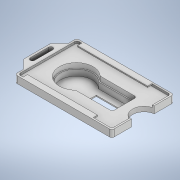
# Autodesk Inventor part: Badge
Saved by Autodesk Inventor 2020 (Build 240168000, 168)
## iProperties
Created: 2019-12-22
Part Number: Badge
Material: Generic
Document SubType Name: Modeling
Designer: user
Density: 1 g/cm^3
Appearance: Default
Author: user
## iProperties of the stored document _3DPrint.ipt
Created: 2019-12-23
Part Number: _3DPrint
Material: Generic
Document SubType Name: Modeling
Designer: user
Density: 1 g/cm^3
Appearance: Default
Author: user
Autodesk Inventor part; units mm, degrees
ref_plane "YZ Plane" through (0, 0, 0) normal (1, 0, 0) x (0, 1, 0)
ref_plane "XZ Plane" through (0, 0, 0) normal (0, 1, 0) x (-1, 0, 0)
ref_plane "XY Plane" through (0, 0, 0) normal (0, 0, 1) x (1, 0, 0)
sketch "Sketch1" plane through (0, 0, 0) normal (0, 1, 0) x (-1, 0, 0)
  line L0 (8.4719, 24.6226) -> (-76.3226, 24.6226)
  line L1 (-76.3281, -32.1774) -> (8.4719, -32.1774)
  line L2 (10.4719, 16.6226) -> (17.8861, 9.2084)
  line L3 (18.4719, 7.7942) -> (18.4719, -15.3489)
  line L4 (17.8861, -16.7632) -> (10.4719, -24.1774)
  line L5 (12.4719, 4.6226) -> (12.4719, -12.1774)
  line L6 (16.4719, -12.1774) -> (16.4719, 4.6226)
  arc A0 (14.4719, -14.1774) -> (16.4719, -12.1774) centre (14.4719, -12.1774) ccw
  arc A1 (12.4719, -12.1774) -> (14.4719, -14.1774) centre (14.4719, -12.1774) ccw
  arc A2 (14.4719, 6.6226) -> (12.4719, 4.6226) centre (14.4719, 4.6226) ccw
  arc A3 (16.4719, 4.6226) -> (14.4719, 6.6226) centre (14.4719, 4.6226) ccw
  arc A4 (-78.3281, -14.1774) -> (-78.3226, 6.6226) centre (-79.4686, -3.7771) ccw
  circle A5 centre (-17.3753, -3.7774) radius 15.5
  line L7 (-61.5377, 5.4726) -> (-61.5377, -13.0274)
  line L8 (-59.5377, -15.0274) -> (-28.0377, -15.0274)
  line L9 (-28.0377, 7.4726) -> (-59.5377, 7.4726)
  arc A6 (-61.5377, -13.0274) -> (-59.5377, -15.0274) centre (-59.5377, -13.0274) ccw
  arc A7 (-59.5377, 7.4726) -> (-61.5377, 5.4726) centre (-59.5377, 5.4726) ccw
  line L10 (-31.4377, 0.4726) -> (-56.9377, 0.4726)
  line L11 (-56.9377, 0.4726) -> (-56.9377, -8.0274)
  line L12 (-56.9377, -8.0274) -> (-31.4377, -8.0274)
  line L13 (-31.4377, -8.0274) -> (-31.4377, 0.4726)
  line L14 (-78.3226, 6.6226) -> (-78.3226, 22.6226)
  line L15 (-78.3281, -14.1774) -> (-78.3281, -30.1774)
  line L16 (6.9737, 23.1226) -> (-74.8281, 23.1226)
  line L17 (-74.8281, -30.6774) -> (6.9737, -30.6774)
  line L18 (8.9737, -28.6774) -> (8.9737, 21.1226)
  line L19 (-76.8281, 21.1226) -> (-76.8281, 6.3469)
  line L20 (-76.8281, -28.6774) -> (-76.8281, -13.901)
  line L21 (10.4719, 22.6226) -> (10.4719, 16.6226)
  line L22 (10.4719, -24.1774) -> (10.4719, -30.1774)
  arc A8 (-78.3281, -30.1774) -> (-76.3281, -32.1774) centre (-76.3281, -30.1774) ccw
  arc A9 (-76.8281, -28.6774) -> (-74.8281, -30.6774) centre (-74.8281, -28.6774) ccw
  arc A10 (-74.8281, 23.1226) -> (-76.8281, 21.1226) centre (-74.8281, 21.1226) ccw
  arc A11 (-76.3226, 24.6226) -> (-78.3226, 22.6226) centre (-76.3226, 22.6226) ccw
  arc A12 (10.4719, 22.6226) -> (8.4719, 24.6226) centre (8.4719, 22.6226) ccw
  arc A13 (8.9737, 21.1226) -> (6.9737, 23.1226) centre (6.9737, 21.1226) ccw
  arc A14 (6.9737, -30.6774) -> (8.9737, -28.6774) centre (6.9737, -28.6774) ccw
  arc A15 (8.4719, -32.1774) -> (10.4719, -30.1774) centre (8.4719, -30.1774) ccw
  arc A16 (17.8861, -16.7632) -> (18.4719, -15.3489) centre (16.4719, -15.3489) ccw
  arc A17 (18.4719, 7.7942) -> (17.8861, 9.2084) centre (16.4719, 7.7942) ccw
  point P0 (0, 0)
  point P1 (10.4719, 24.6226)
  point P2 (-78.3281, -32.1774)
  point P3 (-78.3226, 24.6226)
  point P4 (10.4719, -32.1774)
  point P5 (18.4719, -16.1774)
  point P6 (-61.5377, -15.0274)
  point P7 (14.4719, 6.6226)
  point P8 (14.4719, -14.1774)
  dimension "d0" = 56.8
  dimension "d1" = 88.8
  dimension "d2" = 8
  dimension "d9" = 8
  dimension "d10" = 8
  dimension "d11" = 10
  dimension "d12" = 10
  dimension "d14" = 2
  dimension "d16" = 2
  dimension "d17" = 2
  dimension "d18" = 18
  dimension "d19" = 18
  dimension "d20" = 31
  dimension "d21" = 28.4
  dimension "d22" = 28.4
  dimension "d23" = 20.8
  dimension "d24" = 33.5
  dimension "d25" = 22.5
  dimension "d26" = 2
  dimension "d28" = 7
  dimension "d32" = 7
  dimension "d33" = 4.6
  dimension "d34" = 25.5
  dimension "d36" = 1.5
  dimension "d37" = 1.5
  dimension "d40" = 1.5
  dimension "d41" = 2
  dimension "d76" = 53.8
  dimension "d77" = 15.65
  dimension "d78" = 15.65
  constraints: 46 end point, 38 point on circle, 28 tangent, 18 centre point, 13 point on line, 12 equal radius, 7 parallel, 5 vertical, 3 horizontal, 3 perpendicular, 2 coincident, 1 collinear, 8 other
  measures "d0" distance of point (10.472, -32.177) point (10.472, 24.623)
  measures "d1" distance of point (-78.328, -32.177) point (10.472, -32.177)
  measures "d2" horizontal distance of point (18.472, -16.177) L4.end
  measures "d9" distance of point (10.472, 24.623) L2.start
  measures "d10" distance of point (10.472, -32.177) L4.end
  measures "d14" distance between parallel lines of L3 L6
  measures "d16" radius of A0
  measures "d17" radius of A1
  measures "d18" distance of point (-78.328, -32.177) L15.start
  measures "d19" distance of point (-78.323, 24.623) L14.start
  measures "d20" diameter of A5
  measures "d21" distance from line of L1 A5.centre
  measures "d22" distance from line of L0 A5.centre
  measures "d23" distance of L15.start L14.start
  measures "d24" distance of point (-61.538, -15.027) L8.end
  measures "d25" distance of L8.end L9.start
  measures "d26" radius of A6
  measures "d28" distance between parallel lines of L8 L12
  measures "d32" distance between parallel lines of L10 L9
  measures "d33" distance between parallel lines of L7 L11
  measures "d34" distance of L11.end L12.end
  measures "d36" distance between parallel lines of L0 L16
  measures "d37" distance between parallel lines of L1 L17
  measures "d40" distance between parallel lines of L15 L20
  measures "d41" radius of A8
  measures "d76" distance between parallel lines of L17 L16
  measures "d77" distance between parallel lines of L9 L16
  measures "d78" distance between parallel lines of L17 L8
extrude "OutsideFrame_Ex" add sketch "Sketch1" along normal blind 6.4 contours A12 L21 L2 A17 L3 A16 L4 L22 A15 L1 A8 L15 A4 L20 A9 L17 A14 L18 A13 L16 A10 L19 L14 A11 L0
extrude "CardRidge" add sketch "Sketch1" along normal blind 4.4 contours L19 A10 L16 A13 L18 A14 L17 A9 L20 A4
extrude "TokenBuffer" add sketch "Sketch1" against normal blind 6.6 contours A5 L12 L13 L10 | A5 L10 L11 L12 L8 A6 L7 A7 L9 picked at (-21.5836, -3.7774)
sketch "Sketch4" plane through (0, 0, 0) normal (0, 1, 0) x (1, 0, 0)
  arc A0 (28.0377, 15.0274) -> (28.0377, -7.4726) centre (17.3753, 3.7774) ccw projected
  circle A1 centre (17.3753, 3.7774) radius 14.5
  line L0 (27.6314, -6.4726) -> (60.5377, -6.4726)
  line L1 (60.5377, -6.4726) -> (60.5377, 14.0274)
  line L2 (60.5377, 14.0274) -> (27.6314, 14.0274)
  line L3 (27.6314, 14.0274) -> (27.6314, -6.4726)
  line L4 (59.5377, -7.4726) -> (28.0377, -7.4726) projected
  line L5 (28.0377, 15.0274) -> (59.5377, 15.0274) projected
  line L6 (61.5377, 13.0274) -> (61.5377, -5.4726) projected
  point P0 (0, 0)
  point P1 (27.6314, 14.0274)
  dimension "d56" = 1
  dimension "d57" = 1
  dimension "d58" = 1
  dimension "d59" = 1
  constraints: 8 end point, 2 parallel, 1 coincident, 1 horizontal, 1 perpendicular, 3 other
  measures "d57" distance between parallel lines of L4 L0
  measures "d58" distance between parallel lines of L5 L2
  measures "d59" distance between parallel lines of L6 L1
extrude "TokenCut" cut sketch "Sketch4" against normal blind 5.6
sketch "Sketch5" plane through (74.8281, 6.4, 23.1226) normal (0, 0, -1) x (-1, 0, 0)
  line L0 (-2, 0) -> (0, 0) projected
  line L1 (79.3018, 0) -> (79.3018, -1)
  line L2 (0, 0) -> (81.8018, 0) projected
  line L3 (15, 0) -> (79.3018, 0)
  line L4 (79.3018, 0) -> (79.3018, -1)
  line L5 (79.3018, -1) -> (15, -1)
  line L6 (15, -1) -> (15, 0)
  line L7 (0, -2) -> (0, 0) projected
  line L8 (81.8018, -2) -> (81.8018, 0) projected
  line L9 (0, -2) -> (81.8018, -2) projected
  point P0 (74.8281, -6.4)
  dimension "d65" = 15
  dimension "d66" = 2.5
  dimension "d67" = 1
  constraints: 10 end point, 2 parallel, 1 horizontal, 1 perpendicular, 1 point on line
  measures "d65" distance between parallel lines of L7 L6
  measures "d66" distance between parallel lines of L8 L1
  measures "d67" distance between parallel lines of L5 L2
extrude "LeftSlider" add sketch "Sketch5" along normal blind 4 contours L1 L5 L6 L2
sketch "Sketch6" plane through (-6.9737, 6.4, -30.6774) normal (0, 0, 1) x (1, 0, 0)
  line L0 (83.3018, 0) -> (-1.4982, 0) projected
  line L1 (2.5, 0) -> (66.8018, 0)
  line L2 (66.8018, 0) -> (66.8018, -1)
  line L3 (66.8018, -1) -> (2.5, -1)
  line L4 (2.5, -1) -> (2.5, 0)
  line L5 (0, -2) -> (0, 0) projected
  line L6 (81.8018, -2) -> (81.8018, 0) projected
  point P0 (6.9737, -6.4)
  dimension "d71" = 2.5
  dimension "d72" = 15
  dimension "d73" = 1
  constraints: 8 end point, 2 parallel, 1 horizontal, 1 perpendicular, 1 point on line
  measures "d71" distance between parallel lines of L5 L4
  measures "d72" distance between parallel lines of L6 L2
  measures "d73" distance between parallel lines of L3 L0
extrude "RightSlider" add sketch "Sketch6" along normal blind 4
equation "\"d10\" = d9"
equation "\"d12\" = d11"
equation "\"d18\" = d19"
equation "\"d77\" = d78"
body "Solid3"
